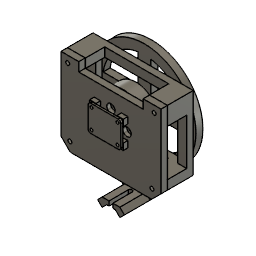
モータ取り付け台 (Autodesk Fusion 360 design; units mm, degrees)
Autodesk Fusion 360 part; units mm, degrees
sketch "スケッチ1" plane through (0, 0, 0) normal (0, 0, 1) x (1, 0, 0)
  line L0 (-38.8909, 38.8909) -> (0, 0)
  line L1 (0, 0) -> (38.8909, 38.8909)
  line L2 (38.8909, 38.8909) -> (-38.8909, 38.8909) construction
  line L3 (0, 38.8909) -> (0, 0) construction
  line L4 (-24.5921, 31.6632) -> (-3.3789, 10.45)
  line L5 (-3.3789, 10.45) -> (3.3789, 10.45)
  line L6 (3.3789, 10.45) -> (24.5921, 31.6632)
  line L7 (24.5921, 31.6632) -> (24.5921, 38.8909)
  line L8 (-24.5921, 38.8909) -> (-24.5921, 31.6632)
  line L9 (-24.5921, 38.8909) -> (24.5921, 38.8909)
  line L10 (-38.8909, 38.8909) -> (-38.8909, 45.9909)
  line L11 (-31.8909, 45.9909) -> (31.8909, 45.9909)
  line L12 (38.8909, 45.9909) -> (38.8909, 38.8909)
  line L13 (31.8909, 45.9909) -> (-31.8909, 45.9909)
  line L14 (-38.8909, 45.9909) -> (-38.8909, 95.9909)
  line L15 (-38.8909, 95.9909) -> (38.8909, 95.9909)
  line L16 (38.8909, 95.9909) -> (38.8909, 45.9909)
  line L17 (38.8909, 45.9909) -> (-38.8909, 95.9909) construction
  line L18 (-38.8909, 45.9909) -> (38.8909, 95.9909) construction
  line L19 (-31.8909, 45.9909) -> (-31.8909, 81.9198)
  line L20 (-24.8198, 88.9909) -> (24.8198, 88.9909)
  line L21 (31.8909, 81.9198) -> (31.8909, 45.9909)
  line L22 (-24.8198, 88.9909) -> (-31.8909, 81.9198)
  line L23 (24.8198, 88.9909) -> (31.8909, 81.9198)
  point P0 (0, 70.9909)
  point P1 (0, 70.9909)
  dimension "d1" = 55
  dimension "d3" = 55
  dimension "d4" = 5
  dimension "d5" = 5
  dimension "d6" = 30
  dimension "d7" = 30
  dimension "d8" = 10.45
  dimension "d9" = 7.1
  dimension "d10" = 50
  dimension "d11" = 7
  dimension "d13" = 45
  dimension "d14" = 45
  dimension "d15" = 10
  dimension "d16" = 10
  dimension "d17" = 7
  dimension "d18" = 7
  dimension "d19" = 57.1
  dimension "d20" = 7.1
  constraint coincident L0.end L1.start
  constraint horizontal L2
  constraint midpoint L2 L3.start
  constraint perpendicular L3 L5
  constraint parallel L0 L4
  constraint parallel L1 L6
  constraint perpendicular L0 L1
  constraint vertical L8
  constraint vertical L7
  constraint coincident L2 L8.start
  constraint coincident L2 L7.end
  constraint coincident L0.start L2.end
  constraint horizontal L11
  constraint vertical L10
  constraint vertical L12
  constraint horizontal L13
  constraint perpendicular L13 L14
  constraint parallel L13 L15
  constraint parallel L14 L16
  constraint coincident L17 P1
  constraint coincident L18 P1
  constraint coincident L10.end L14.start
  constraint coincident P1 P0
  measures "d1" distance of L0.end L1.end
  measures "d3" distance of L0.start L0.end
  measures "d4" distance of L1 L6
  measures "d5" distance of L0 L4
  measures "d6" distance of L5.end L6.end
  measures "d7" distance of L4.start L4.end
  measures "d8" distance of L0.end L5
  measures "d9" distance of L9 L11
  measures "d10" distance of L12.start L15.end
  measures "d11" distance of L16 L21
  measures "d13" angle of L20 L22
  measures "d14" angle of L20 L23
  measures "d15" distance of L20.start L19.end
  measures "d16" distance of L20.end L21.start
  measures "d17" distance of L15 L20
  measures "d18" distance of L14 L19
  measures "d19" distance of L9 L15
  measures "d20" distance of L0.start L10.end
extrude "押し出し1" add sketch "スケッチ1" along normal mid plane 5 makes body 1
sketch "スケッチ2" plane through (0, 0, 2.5) normal (0, 0, 1) x (1, 0, 0)
  line L0 (-31.8909, 81.9198) -> (-24.8198, 88.9909)
  line L1 (-24.8198, 88.9909) -> (24.8198, 88.9909)
  line L2 (24.8198, 88.9909) -> (31.8909, 81.9198)
  line L3 (31.8909, 81.9198) -> (31.8909, 45.9909)
  line L4 (31.8909, 45.9909) -> (-31.8909, 45.9909)
  line L5 (-31.8909, 45.9909) -> (-31.8909, 81.9198)
  line L6 (-3.3789, 10.45) -> (-24.5921, 31.6632)
  line L7 (-24.5921, 31.6632) -> (-24.5921, 38.8909)
  line L8 (-24.5921, 38.8909) -> (24.5921, 38.8909)
  line L9 (24.5921, 38.8909) -> (24.5921, 31.6632)
  line L10 (24.5921, 31.6632) -> (3.3789, 10.45)
  line L11 (3.3789, 10.45) -> (-3.3789, 10.45)
  line L12 (-38.8909, 38.8909) -> (0, 0)
  line L13 (0, 0) -> (38.8909, 38.8909)
  line L14 (38.8909, 38.8909) -> (38.8909, 95.9909)
  line L15 (38.8909, 95.9909) -> (-38.8909, 95.9909)
  line L16 (-38.8909, 95.9909) -> (-38.8909, 38.8909)
  line L17 (-24.8198, 95.9909) -> (-24.8198, 88.9909)
  line L18 (-24.8198, 88.9909) -> (-31.8909, 81.9198)
  line L19 (-31.8909, 81.9198) -> (-38.8909, 81.9198)
  line L20 (-38.8909, 81.9198) -> (-38.8909, 95.9909)
  line L21 (-38.8909, 95.9909) -> (-24.8198, 95.9909)
  line L22 (24.8198, 95.9909) -> (24.8198, 88.9909)
  line L23 (24.8198, 88.9909) -> (31.8909, 81.9198)
  line L24 (31.8909, 81.9198) -> (38.8909, 81.9198)
  line L25 (38.8909, 81.9198) -> (38.8909, 95.9909)
  line L26 (38.8909, 95.9909) -> (24.8198, 95.9909)
  line L27 (-24.5921, 45.9909) -> (-24.5921, 31.6632)
  line L28 (-24.5921, 31.6632) -> (-31.6632, 31.6632)
  line L29 (-31.6632, 31.6632) -> (-38.8909, 38.8909)
  line L30 (-38.8909, 38.8909) -> (-38.8909, 45.9909)
  line L31 (-38.8909, 45.9909) -> (-24.5921, 45.9909)
  line L32 (24.5921, 45.9909) -> (24.5921, 31.6632)
  line L33 (24.5921, 31.6632) -> (31.6632, 31.6632)
  line L34 (31.6632, 31.6632) -> (38.8909, 38.8909)
  line L35 (38.8909, 38.8909) -> (38.8909, 45.9909)
  line L36 (38.8909, 45.9909) -> (24.5921, 45.9909)
  line L37 (-3.3789, 10.45) -> (-6.9145, 6.9145)
  line L38 (-6.9145, 6.9145) -> (0, 0)
  line L39 (0, 0) -> (6.9145, 6.9145)
  line L40 (6.9145, 6.9145) -> (3.3789, 10.45)
  line L41 (3.3789, 10.45) -> (-3.3789, 10.45)
  constraint coincident L15 L17.start
  constraint coincident L0.end L1.start
  constraint perpendicular L1 L17
  constraint coincident L0.start L5.end
  constraint coincident L16 L19.end
  constraint perpendicular L16 L19
  constraint coincident L15.end L16.start
  constraint coincident L15 L22.start
  constraint coincident L1.end L2.start
  constraint coincident L2.end L3.start
  constraint coincident L14 L24.end
  constraint perpendicular L14 L24
  constraint coincident L14.end L15.start
  constraint vertical L22
  constraint coincident L4 L27.start
  constraint coincident L6.end L7.start
  constraint coincident L12 L28.end
  constraint perpendicular L27 L28
  constraint vertical L27
  constraint coincident L16 L30.end
  constraint coincident L12.start L16.end
  constraint horizontal L31
  constraint vertical L32
  constraint perpendicular L32 L33
  constraint perpendicular L33 L35
  constraint coincident L4 L32.start
  constraint coincident L9.end L10.start
  constraint coincident L13 L33.end
  constraint coincident L14 L35.end
  constraint coincident L13.end L14.start
  constraint horizontal L36
  constraint coincident L6.start L11.end
  constraint coincident L12 L37.end
  constraint perpendicular L12 L37
  constraint perpendicular L12 L39
  constraint coincident L10.end L11.start
  constraint coincident L13 L39.end
  constraint coincident L12.end L13.start
  constraint perpendicular L13 L40
extrude "押し出し2" add sketch "スケッチ2" along normal blind 15 contours L0 L15 L16 L17 L18 L19 L20 L21 | L4 L7 L12 L16 L27 L28 L29 L30 L31 | L2 L14 L15 L22 L23 L24 L25 L26 | L4 L9 L13 L14 L32 L33 L34 L35 L36 bodies 1
extrude "押し出し3" add sketch "スケッチ2" along normal blind 60 contours L11 L12 L13 L37 L38 L39 L40 L41 bodies 1
sketch "スケッチ3" plane through (0, 0, -2.5) normal (0, 0, -1) x (-1, 0, 0)
  line L0 (24.8198, 88.9909) -> (31.8909, 81.9198)
  line L1 (31.8909, 81.9198) -> (31.8909, 45.9909)
  line L2 (31.8909, 45.9909) -> (-31.8909, 45.9909)
  line L3 (-31.8909, 45.9909) -> (-31.8909, 81.9198)
  line L4 (-31.8909, 81.9198) -> (-24.8198, 88.9909)
  line L5 (-24.8198, 88.9909) -> (24.8198, 88.9909)
  line L6 (24.5921, 31.6632) -> (3.3789, 10.45)
  line L7 (3.3789, 10.45) -> (-3.3789, 10.45)
  line L8 (-3.3789, 10.45) -> (-24.5921, 31.6632)
  line L9 (-24.5921, 31.6632) -> (-24.5921, 38.8909)
  line L10 (-24.5921, 38.8909) -> (24.5921, 38.8909)
  line L11 (24.5921, 38.8909) -> (24.5921, 31.6632)
  line L12 (0, 0) -> (38.8909, 38.8909)
  line L13 (38.8909, 38.8909) -> (38.8909, 95.9909)
  line L14 (38.8909, 95.9909) -> (-38.8909, 95.9909)
  line L15 (-38.8909, 95.9909) -> (-38.8909, 38.8909)
  line L16 (-38.8909, 38.8909) -> (0, 0)
  line L17 (-38.8909, 95.9909) -> (-28.3553, 85.4553) construction
  line L18 (38.8909, 95.9909) -> (28.3553, 85.4553) construction
  circle A0 centre (-33.6231, 90.7231) radius 3.5
  circle A1 centre (33.6231, 90.7231) radius 3.5
  circle A2 centre (-31.8909, 38.8909) radius 3.5
  circle A3 centre (31.8909, 38.8909) radius 3.5
  line L19 (-24.5921, 38.8909) -> (-38.8909, 38.8909) construction
  line L20 (-31.8909, 45.9909) -> (-31.8909, 31.8909) construction
  line L21 (24.5921, 38.8909) -> (38.8909, 38.8909) construction
  line L22 (31.8909, 45.9909) -> (31.8909, 31.8909) construction
  circle A4 centre (-31.8909, 38.8909) radius 1.5
  circle A5 centre (31.8909, 38.8909) radius 1.5
  circle A6 centre (33.6231, 90.7231) radius 1.5
  circle A7 centre (-33.6231, 90.7231) radius 1.5
  dimension "d27" = 7
  dimension "d28" = 7
  dimension "d29" = 7
  dimension "d30" = 7
  dimension "d31" = 3
  dimension "d32" = 3
  dimension "d33" = 3
  dimension "d34" = 3
  constraint coincident L14.end L15.start
  constraint midpoint L4 L17.end
  constraint coincident L13.end L14.start
  constraint midpoint L0 L18.end
  constraint midpoint L17 A0.centre
  constraint midpoint L18 A1.centre
  constraint coincident L9.end L10.start
  constraint coincident L15.end L16.start
  constraint coincident L2.end L3.start
  constraint coincident L16 L20.end
  constraint perpendicular L19 L20
  constraint coincident A2.centre L19
  constraint coincident A2.centre L20
  constraint coincident L10.end L11.start
  constraint coincident L12.end L13.start
  constraint coincident L1.end L2.start
  constraint coincident L12 L22.end
  constraint perpendicular L21 L22
  constraint coincident A3.centre L22
  constraint coincident A3.centre L21
  constraint concentric A2 A4
  constraint concentric A3 A5
  constraint concentric A1 A6
  constraint concentric A0 A7
  measures "d27" diameter of A0
  measures "d28" diameter of A1
  measures "d29" diameter of A2
  measures "d30" diameter of A3
  measures "d31" diameter of A4
  measures "d32" diameter of A5
  measures "d33" diameter of A6
  measures "d34" diameter of A7
extrude "押し出し4" cut sketch "スケッチ3" against normal blind 25 contours A4 | A5 | A6 | A7 bodies 1
extrude "押し出し7" cut 1 faces at (0, 6.9667, 62.5) along direction (0, 0, -1) blind 65 on bodies 1 bodies 1
sketch "スケッチ8" plane through (0, 0, 2.5) normal (0, 0, 1) x (1, 0, 0)
  line L0 (-6.9145, 6.9145) -> (-3.3789, 10.45)
  line L1 (-3.3789, 10.45) -> (-24.5921, 31.6632)
  line L2 (-24.5921, 31.6632) -> (-31.6632, 31.6632)
  line L3 (-31.6632, 31.6632) -> (-6.9145, 6.9145)
  line L4 (3.3789, 10.45) -> (6.9145, 6.9145)
  line L5 (24.5921, 31.6632) -> (3.3789, 10.45)
  line L6 (6.9145, 6.9145) -> (31.6632, 31.6632)
  line L7 (-3.3789, 10.45) -> (3.3789, 10.45)
  line L8 (-6.9145, 13.9855) -> (6.9145, 13.9855)
  line L9 (6.9145, 13.9855) -> (10.45, 10.45)
  line L10 (-6.9145, 13.9855) -> (-10.45, 10.45)
  dimension "d52" = 5
  dimension "d53" = 5
  constraint coincident L0.end L1.start
  constraint coincident L4.start L5.end
  constraint coincident L1 L8.start
  constraint coincident L5 L8.end
  constraint coincident L6 L9.end
  constraint coincident L3 L10.end
  constraint perpendicular L1 L10
  constraint perpendicular L6 L9
  measures "d52" distance of L0 L10
  measures "d53" distance of L4 L9
extrude "押し出し9" add sketch "スケッチ8" against normal blind 5 contours L1 L5 L7 L8 bodies 1
extrude "押し出し10" add sketch "スケッチ8" along normal blind 20 contours L0 L1 L3 L10 | L1 L5 L7 L8 | L4 L5 L6 L9 bodies 1
sketch "スケッチ9" plane through (0, 10.45, 0) normal (0, -1, 0) x (1, 0, 0)
  line L0 (-3.3789, 22.5) -> (-3.3789, -2.5)
  line L1 (-3.3789, -2.5) -> (3.3789, -2.5)
  line L2 (3.3789, -2.5) -> (3.3789, 22.5)
  line L3 (3.3789, 22.5) -> (-3.3789, 22.5)
  arc A0 (-1.5, 7.5) -> (1.5, 7.5) centre (0, 7.5) ccw
  line L4 (0, 7.5) -> (0, -2.5) construction
  line L5 (-1.5, 7.5) -> (-1.5, 22.5)
  line L6 (1.5, 22.5) -> (1.5, 7.5)
  dimension "d58" = 10
  dimension "d59" = 1.5
  constraint coincident A0.centre L4.start
  constraint midpoint L1 L4.end
  constraint vertical L4
  constraint coincident L3 L5.end
  constraint tangent A0 L5
  constraint coincident L3 L6.start
  constraint tangent A0 L6
  constraint vertical L6
  constraint vertical L5
  measures "d58" distance of A0.centre L4.end
  measures "d59" radius of A0
extrude "押し出し11" cut sketch "スケッチ9" against normal blind 4 contours L3 A0 L5 L6 bodies 1
extrude "押し出し12" add sketch "スケッチ3" against normal blind 4 contours A4 | A5 | A6 | A7 bodies 1
sketch "スケッチ10" plane through (0, 0, 17.5) normal (0, 0, 1) x (1, 0, 0)
  circle A0 centre (-31.8909, 38.8909) radius 1.5
  line L0 (-38.8909, 45.9909) -> (-38.8909, 38.8909)
  line L1 (-38.8909, 38.8909) -> (-31.6632, 31.6632)
  line L2 (-31.6632, 31.6632) -> (-24.5921, 31.6632)
  line L3 (-24.5921, 31.6632) -> (-24.5921, 45.9909)
  line L4 (-24.5921, 45.9909) -> (-38.8909, 45.9909)
  line L5 (-38.8909, 95.9909) -> (-38.8909, 81.9198)
  line L6 (31.6632, 31.6632) -> (38.8909, 38.8909)
  line L7 (38.8909, 81.9198) -> (38.8909, 95.9909)
  line L8 (-38.8909, 95.9909) -> (-38.8909, 38.8909)
  line L9 (-38.8909, 38.8909) -> (-31.6632, 31.6632)
  line L10 (-31.6632, 31.6632) -> (31.6632, 31.6632)
  line L11 (31.6632, 31.6632) -> (38.8909, 38.8909)
  line L12 (38.8909, 38.8909) -> (38.8909, 95.9909)
  line L13 (38.8909, 95.9909) -> (-38.8909, 95.9909)
  line L14 (31.8909, 45.9909) -> (31.8909, 81.9198)
  line L15 (31.8909, 81.9198) -> (24.8198, 88.9909)
  line L16 (6.9145, 13.9855) -> (24.5921, 31.6632)
  line L17 (24.5921, 31.6632) -> (24.5921, 38.8909)
  line L18 (24.5921, 38.8909) -> (-24.5921, 38.8909)
  line L19 (-24.5921, 38.8909) -> (-24.5921, 31.6632)
  line L20 (-24.5921, 31.6632) -> (-6.9145, 13.9855)
  line L21 (-6.9145, 13.9855) -> (6.9145, 13.9855)
  line L22 (3.3789, 10.45) -> (-3.3789, 10.45)
  line L23 (-3.3789, 10.45) -> (-6.9145, 6.9145)
  line L24 (-6.9145, 6.9145) -> (-38.8909, 38.8909)
  line L25 (-38.8909, 38.8909) -> (-38.8909, 95.9909)
  line L26 (-38.8909, 95.9909) -> (38.8909, 95.9909)
  line L27 (38.8909, 95.9909) -> (38.8909, 38.8909)
  line L28 (38.8909, 38.8909) -> (6.9145, 6.9145)
  line L29 (6.9145, 6.9145) -> (3.3789, 10.45)
  line L30 (-24.8198, 88.9909) -> (-31.8909, 81.9198)
  line L31 (-31.8909, 81.9198) -> (-31.8909, 45.9909)
  line L32 (-31.8909, 45.9909) -> (31.8909, 45.9909)
  line L33 (31.8909, 45.9909) -> (31.8909, 81.9198)
  line L34 (31.8909, 81.9198) -> (24.8198, 88.9909)
  line L35 (24.8198, 88.9909) -> (-24.8198, 88.9909)
  line L36 (0, 88.9909) -> (0, 45.9909) construction
  circle A1 centre (0, 76.9909) radius 1.5
  circle A2 centre (12.5, 67.4909) radius 1.5
  circle A3 centre (0, 57.9909) radius 1.5
  circle A4 centre (-12.5, 67.4909) radius 1.5
  line L37 (-12.5, 67.4909) -> (12.5, 67.4909) construction
  line L38 (0, 76.9909) -> (0, 57.9909) construction
  circle A5 centre (31.8909, 38.8909) radius 1.5
  circle A6 centre (33.6231, 90.7231) radius 1.5
  circle A7 centre (-33.6231, 90.7231) radius 1.5
  circle A8 centre (-33.6231, 90.7231) radius 1.5
  circle A9 centre (33.6231, 90.7231) radius 1.5
  circle A10 centre (31.8909, 38.8909) radius 1.5
  circle A11 centre (0, 67.4909) radius 4
  point P0 (0, 67.4909)
  dimension "d64" = 3
  dimension "d65" = 3
  dimension "d66" = 3
  dimension "d67" = 3
  dimension "d68" = 19
  dimension "d69" = 25
  dimension "d70" = 12.5
  dimension "d71" = 9.5
  dimension "d78" = 3
  dimension "d79" = 3
  dimension "d80" = 3
  dimension "d81" = 8
  constraint coincident L5.start L8.start
  constraint coincident L0.end L1.start
  constraint coincident L1.end L2.start
  constraint coincident L6.start L10.end
  constraint coincident L6.end L11.end
  constraint coincident L7.end L12.end
  constraint midpoint L35 L36.start
  constraint midpoint L32 L36.end
  constraint midpoint L36 P0
  constraint coincident A4.centre L37.start
  constraint coincident A2.centre L37.end
  constraint coincident A1.centre L38.start
  constraint coincident A3.centre L38.end
  constraint coincident P0 L37
  constraint coincident P0 L38
  constraint vertical L38
  constraint horizontal L37
  constraint concentric A7 A8
  constraint concentric A6 A9
  constraint concentric A5 A10
  constraint coincident P0 A11.centre
  measures "d64" diameter of A1
  measures "d65" diameter of A3
  measures "d66" diameter of A4
  measures "d67" diameter of A2
  measures "d68" distance of A1.centre A3.centre
  measures "d69" distance of A2.centre A4.centre
  measures "d70" distance of P0 A2.centre
  measures "d71" distance of P0 A1.centre
  measures "d78" diameter of A10
  measures "d79" diameter of A9
  measures "d80" diameter of A8
  measures "d81" diameter of A11
extrude "押し出し13" add sketch "スケッチ10" along normal blind 5 separate body contours L0 L1 L2 L3 L4 L8 L9 L10 L19 L24 L25 L32 | L3 L4 L5 L6 L7 L8 L10 L11 L12 L13 L14 L15 L17 L18 L25 L26 L27 L28 L30 L31 L32 L33 L34 L35 | L4 L14 L15 L30 L31 L32 L33 L34 L35 | L3 L10 L17 L18 L19 makes body 2
sketch "スケッチ11" plane through (0, 0, 22.5) normal (0, 0, 1) x (1, 0, 0)
  circle A0 centre (-12.5, 67.4909) radius 1.5
  circle A1 centre (0, 76.9909) radius 1.5
  circle A2 centre (0, 57.9909) radius 1.5
  circle A3 centre (12.5, 67.4909) radius 1.5
  line L0 (-31.6632, 31.6632) -> (31.6632, 31.6632)
  line L1 (31.6632, 31.6632) -> (38.8909, 38.8909)
  line L2 (38.8909, 38.8909) -> (38.8909, 95.9909)
  line L3 (38.8909, 95.9909) -> (-38.8909, 95.9909)
  line L4 (-38.8909, 95.9909) -> (-38.8909, 38.8909)
  line L5 (-38.8909, 38.8909) -> (-31.6632, 31.6632)
  line L6 (25, 95.9909) -> (-25, 95.9909)
  line L7 (-25, 95.9909) -> (-25, 88.9909)
  line L8 (-25, 88.9909) -> (25, 88.9909)
  line L9 (25, 88.9909) -> (25, 95.9909)
  line L10 (25, 95.9909) -> (-25, 88.9909) construction
  line L11 (-25, 95.9909) -> (25, 88.9909) construction
  line L12 (0, 76.9909) -> (0, 92.4909) construction
  circle A4 centre (-31.8909, 38.8909) radius 1.5
  circle A5 centre (31.8909, 38.8909) radius 1.5
  circle A6 centre (33.6231, 90.7231) radius 1.5
  circle A7 centre (-33.6231, 90.7231) radius 1.5
  circle A8 centre (0, 67.4909) radius 4
  point P0 (0, 92.4909)
  dimension "d74" = 50
  dimension "d75" = 7
  constraint horizontal L6
  constraint perpendicular L6 L7
  constraint parallel L6 L8
  constraint parallel L7 L9
  constraint coincident L10 P0
  constraint coincident L11 P0
  constraint coincident L3 L6.start
  constraint coincident A1.centre L12.start
  constraint coincident P0 L12.end
  constraint vertical L12
  measures "d74" distance of L7.end L8.end
  measures "d75" distance of L6.start L8.end
extrude "押し出し14" cut sketch "スケッチ11" against normal blind 5 contours L3 L6 L7 L8 L9 bodies 2
sketch "スケッチ12" plane through (0, 0, 17.5) normal (0, 0, -1) x (-1, 0, 0)
  line L0 (25, 95.9909) -> (25, 88.9909)
  line L1 (25, 88.9909) -> (-25, 88.9909)
  line L2 (-25, 88.9909) -> (-25, 95.9909)
  line L3 (-25, 95.9909) -> (-38.8909, 95.9909)
  line L4 (-38.8909, 95.9909) -> (-38.8909, 38.8909)
  line L5 (-38.8909, 38.8909) -> (-31.6632, 31.6632)
  line L6 (-31.6632, 31.6632) -> (31.6632, 31.6632)
  line L7 (31.6632, 31.6632) -> (38.8909, 38.8909)
  line L8 (38.8909, 38.8909) -> (38.8909, 95.9909)
  line L9 (38.8909, 95.9909) -> (25, 95.9909)
  circle A0 centre (-12.5, 67.4909) radius 1.5
  circle A1 centre (0, 57.9909) radius 1.5
  circle A2 centre (33.6231, 90.7231) radius 1.5
  circle A3 centre (0, 67.4909) radius 4
  circle A4 centre (-31.8909, 38.8909) radius 1.5
  circle A5 centre (31.8909, 38.8909) radius 1.5
  circle A6 centre (12.5, 67.4909) radius 1.5
  circle A7 centre (-33.6231, 90.7231) radius 1.5
  circle A8 centre (0, 76.9909) radius 1.5
  circle A9 centre (0, 67.4909) radius 16.25
  dimension "d82" = 32.5
  constraint concentric A3 A9
  measures "d82" diameter of A9
extrude "押し出し15" add sketch "スケッチ12" along normal blind 1.5 separate body contours A9 makes body 3
sketch "スケッチ13" plane through (0, 0, 16) normal (0, 0, -1) x (-1, 0, 0)
  circle A0 centre (0, 76.9909) radius 1.5
  circle A1 centre (0, 67.4909) radius 4
  circle A2 centre (0, 57.9909) radius 1.5
  circle A3 centre (12.5, 67.4909) radius 1.5
  circle A4 centre (-12.5, 67.4909) radius 1.5
  circle A5 centre (0, 67.4909) radius 16.25
  circle A6 centre (0, 67.4909) radius 7.5
  dimension "d85" = 15
  constraint concentric A1 A6
  measures "d85" diameter of A6
extrude "押し出し16" add sketch "スケッチ13" along normal blind 3 contours A6 bodies 3
sketch "スケッチ15" plane through (0, 0, 13) normal (0, 0, -1) x (-1, 0, 0)
  circle A0 centre (0, 67.4909) radius 4
  circle A1 centre (0, 67.4909) radius 7.5
  circle A2 centre (0, 67.4909) radius 17.5
  dimension "d88" = 35
  constraint concentric A0 A2
  measures "d88" diameter of A2
extrude "押し出し17" add sketch "スケッチ15" along normal blind 9 contours A0 | A1 | A2 bodies 3
sketch "スケッチ16" plane through (0, 0, 13) normal (0, 0, 1) x (1, 0, 0)
  circle A0 centre (0, 67.4909) radius 4
  circle A1 centre (0, 67.4909) radius 3.25
  dimension "d91" = 6.5
  constraint concentric A0 A1
  measures "d91" diameter of A1
extrude "押し出し18" add sketch "スケッチ16" along normal blind 7 contours A1 bodies 3
sketch "スケッチ17" plane through (0, 0, 0) normal (1, 0, 0) x (0, 0, -1)
  line L0 (-4, 49.9909) -> (-4, 84.9909)
  line L1 (-4, 84.9909) -> (-3, 84.9909)
  line L2 (-18, 67.4909) -> (2, 67.4909)
  line L3 (-1, 67.4909) -> (-4, 67.4909)
  line L4 (-4, 84.9909) -> (-4, 67.4909)
  line L5 (-20, 70.7409) -> (-20, 64.2409)
  line L6 (-3, 84.9909) -> (-1, 74.4909)
  line L7 (-1, 74.4909) -> (-1, 67.4909)
  dimension "d94" = 19
  dimension "d95" = 1
  dimension "d96" = 7
  constraint coincident L0.end L1.start
  constraint perpendicular L0 L1
  constraint coincident L3.start L2
  constraint midpoint L0 L3.end
  constraint vertical L7
  measures "d94" distance of L3.start L5
  measures "d95" distance of L0.end L1.end
  measures "d96" distance of L3.start L6.end
revolve "回転1" add sketch "スケッチ17" angle 360 about axis through (0, 67.4909, 18) along (0, 0, -1) bodies 3
sketch "スケッチ18" plane through (0, 0, 1) normal (0, 0, -1) x (-1, 0, 0)
  circle A0 centre (0, 67.4909) radius 7
  circle A1 centre (0, 67.4909) radius 2
  dimension "d98" = 4
  constraint concentric A0 A1
  measures "d98" diameter of A1
extrude "押し出し19" add sketch "スケッチ18" along normal blind 9.1 contours A1 bodies 3
sketch "スケッチ19" plane through (0, 0, -2.5) normal (0, 0, -1) x (-1, 0, 0)
  line L0 (-6.9145, 13.9855) -> (-24.5921, 31.6632)
  line L1 (-24.5921, 31.6632) -> (-24.5921, 38.8909)
  line L2 (-24.5921, 38.8909) -> (24.5921, 38.8909)
  line L3 (24.5921, 38.8909) -> (24.5921, 31.6632)
  line L4 (24.5921, 31.6632) -> (6.9145, 13.9855)
  line L5 (6.9145, 13.9855) -> (-6.9145, 13.9855)
  line L6 (-3.3789, 10.45) -> (3.3789, 10.45)
  line L7 (3.3789, 10.45) -> (6.9145, 6.9145)
  line L8 (6.9145, 6.9145) -> (38.8909, 38.8909)
  line L9 (38.8909, 38.8909) -> (38.8909, 95.9909)
  line L10 (38.8909, 95.9909) -> (-38.8909, 95.9909)
  line L11 (-38.8909, 95.9909) -> (-38.8909, 38.8909)
  line L12 (-38.8909, 38.8909) -> (-6.9145, 6.9145)
  line L13 (-6.9145, 6.9145) -> (-3.3789, 10.45)
  line L14 (24.8198, 88.9909) -> (31.8909, 81.9198)
  line L15 (31.8909, 81.9198) -> (31.8909, 45.9909)
  line L16 (31.8909, 45.9909) -> (-31.8909, 45.9909)
  line L17 (-31.8909, 45.9909) -> (-31.8909, 81.9198)
  line L18 (-31.8909, 81.9198) -> (-24.8198, 88.9909)
  line L19 (-24.8198, 88.9909) -> (24.8198, 88.9909)
  circle A0 centre (0, 67.4909) radius 2
  circle A1 centre (0, 67.4909) radius 2
  circle A2 centre (0, 67.4909) radius 40
  circle A3 centre (0, 67.4909) radius 10
  circle A4 centre (0, 67.4909) radius 3.75
  circle A5 centre (0, 67.4909) radius 32.5
  line L20 (-5, 99.604) -> (-5, 76.1511)
  line L21 (5, 99.604) -> (5, 76.1511)
  line L22 (8.6603, 72.4909) -> (32.1131, 72.4909)
  line L23 (8.6603, 62.4909) -> (32.1131, 62.4909)
  line L24 (5, 58.8306) -> (5, 35.3778)
  line L25 (-5, 58.8306) -> (-5, 35.3778)
  line L26 (-8.6603, 62.4909) -> (-32.1131, 62.4909)
  line L27 (-8.6603, 72.4909) -> (-32.1131, 72.4909)
  dimension "d101" = 4
  dimension "d102" = 80
  dimension "d103" = 20
  dimension "d104" = 7.5
  dimension "d107" = 65
  dimension "d108" = 10
  dimension "d109" = 10
  dimension "d110" = 10
  dimension "d111" = 10
  dimension "d112" = 5
  dimension "d113" = 5
  dimension "d114" = 5
  dimension "d115" = 5
  constraint concentric A0 A1
  constraint concentric A0 A2
  constraint concentric A1 A3
  constraint concentric A3 A4
  constraint concentric A1 A5
  constraint coincident A5 L20.start
  constraint coincident A3 L20.end
  constraint perpendicular L19 L20
  constraint coincident A5 L21.start
  constraint coincident A3 L21.end
  constraint perpendicular L19 L21
  constraint coincident A3 L22.start
  constraint coincident A5 L22.end
  constraint perpendicular L15 L22
  constraint coincident A3 L23.start
  constraint coincident A3 L24.start
  constraint coincident A5 L24.end
  constraint perpendicular L2 L24
  constraint coincident A3 L25.start
  constraint coincident A5 L25.end
  constraint coincident A3 L26.start
  constraint coincident A5 L26.end
  constraint coincident A3 L27.start
  constraint coincident A5 L27.end
  constraint coincident A5 L23.end
  constraint horizontal L27
  constraint horizontal L26
  constraint horizontal L23
  constraint vertical L25
  measures "d101" diameter of A1
  measures "d102" diameter of A2
  measures "d103" diameter of A3
  measures "d104" diameter of A4
  measures "d107" diameter of A5
  measures "d108" distance of L22 L23
  measures "d109" distance of L20 L21
  measures "d110" distance of L26 L27
  measures "d111" distance of L24 L25
  measures "d112" distance of A0.centre L27
  measures "d113" distance of A0.centre L21
  measures "d114" distance of A0.centre L22
  measures "d115" distance of A0.centre L24
extrude "押し出し20" add sketch "スケッチ19" against normal blind 3.5 separate body contours A4 makes body 4
extrude "押し出し21" add sketch "スケッチ19" along normal blind 6.5 contours L1 L2 L10 L11 L16 L17 L18 L19 A2 A5 | L1 L2 L3 A2 A5 | L11 A2 | L2 L3 L9 L10 L14 L15 L16 L19 A2 A5 | L9 A2 | L2 L16 L24 L25 | L2 A5 L24 L25 | L16 L17 A5 | L10 A2 A5 | L16 A3 L24 L25 | L15 L16 A5 | A3 | L17 A5 L26 L27 | L17 A3 L26 L27 | L10 A5 L20 L21 | L10 L19 L20 L21 | L17 L18 L19 A5 | L19 A3 L20 L21 | L14 L15 L19 A5 | L15 A3 L22 L23 | L15 A5 L22 L23 | A4 bodies 4
extrude "押し出し22" cut 1 faces at (24.2955, 69.1575, -2.5) along direction (0, 0, -1) blind 1 on bodies 4 bodies 4
sketch "スケッチ20" plane through (0, 0, -9) normal (0, 0, -1) x (-1, 0, 0)
  circle A0 centre (0, 67.4909) radius 2
  line L0 (32.1131, 72.4909) -> (8.6603, 72.4909)
  arc A1 (8.6603, 72.4909) -> (5, 76.1511) centre (0, 67.4909) ccw
  line L1 (5, 76.1511) -> (5, 99.604)
  arc A2 (32.1131, 72.4909) -> (5, 99.604) centre (0, 67.4909) ccw
  arc A3 (-5, 99.604) -> (-32.1131, 72.4909) centre (0, 67.4909) ccw
  line L2 (-5, 99.604) -> (-5, 76.1511)
  arc A4 (-5, 76.1511) -> (-8.6603, 72.4909) centre (0, 67.4909) ccw
  line L3 (-8.6603, 72.4909) -> (-32.1131, 72.4909)
  arc A5 (5, 58.8306) -> (8.6603, 62.4909) centre (0, 67.4909) ccw
  line L4 (8.6603, 62.4909) -> (32.1131, 62.4909)
  arc A6 (5, 35.3778) -> (32.1131, 62.4909) centre (0, 67.4909) ccw
  line L5 (5, 35.3778) -> (5, 58.8306)
  arc A7 (-8.6603, 62.4909) -> (-5, 58.8306) centre (0, 67.4909) ccw
  line L6 (-5, 58.8306) -> (-5, 35.3778)
  arc A8 (-32.1131, 62.4909) -> (-5, 35.3778) centre (0, 67.4909) ccw
  line L7 (-32.1131, 62.4909) -> (-8.6603, 62.4909)
  circle A9 centre (0, 67.4909) radius 40
  circle A10 centre (0, 67.4909) radius 2
  dimension "d120" = 4
  constraint concentric A0 A10
  measures "d120" diameter of A10
extrude "押し出し23" add sketch "スケッチ20" against normal blind 0.9 contours A0 A10 bodies 4
sketch "スケッチ21" plane through (0, 0, 22.5) normal (0, 0, 1) x (1, 0, 0)
  circle A0 centre (12.5, 67.4909) radius 1.5
  circle A1 centre (0, 57.9909) radius 1.5
  circle A2 centre (-33.6231, 90.7231) radius 1.5
  circle A3 centre (0, 67.4909) radius 4
  circle A4 centre (31.8909, 38.8909) radius 1.5
  circle A5 centre (-31.8909, 38.8909) radius 1.5
  circle A6 centre (-12.5, 67.4909) radius 1.5
  circle A7 centre (33.6231, 90.7231) radius 1.5
  circle A8 centre (0, 76.9909) radius 1.5
  line L0 (-25, 88.9909) -> (-25, 95.9909)
  line L1 (-25, 95.9909) -> (-38.8909, 95.9909)
  line L2 (-38.8909, 95.9909) -> (-38.8909, 38.8909)
  line L3 (-38.8909, 38.8909) -> (-31.6632, 31.6632)
  line L4 (-31.6632, 31.6632) -> (31.6632, 31.6632)
  line L5 (31.6632, 31.6632) -> (38.8909, 38.8909)
  line L6 (38.8909, 38.8909) -> (38.8909, 95.9909)
  line L7 (38.8909, 95.9909) -> (25, 95.9909)
  line L8 (25, 95.9909) -> (25, 88.9909)
  line L9 (25, 88.9909) -> (-25, 88.9909)
  circle A9 centre (0, 76.9909) radius 3.25
  circle A10 centre (12.5, 67.4909) radius 3.25
  circle A11 centre (-12.5, 67.4909) radius 3.25
  circle A12 centre (0, 57.9909) radius 3.25
  dimension "d123" = 6.5
  dimension "d124" = 6.5
  dimension "d125" = 6.5
  dimension "d126" = 6.5
  constraint concentric A8 A9
  constraint concentric A0 A10
  constraint concentric A6 A11
  constraint concentric A1 A12
  measures "d123" diameter of A9
  measures "d124" diameter of A10
  measures "d125" diameter of A11
  measures "d126" diameter of A12
extrude "押し出し24" cut sketch "スケッチ21" against normal blind 3 contours A9 | A10 | A11 | A12 bodies 2
ref_plane "作業平面1" through (0, 63.827, 26) normal (0, 0, 1) x (1, 0, 0)
sketch "スケッチ22" plane through (0, 0, 26) normal (0, 0, 1) x (1, 0, 0)
  circle A0 centre (0, 67.4909) radius 3.25
  line L0 (10.7, 57.3309) -> (-10.7, 57.3309)
  line L1 (-12.7, 59.3309) -> (-12.7, 75.6509)
  line L2 (-10.7, 77.6509) -> (10.7, 77.6509)
  line L3 (12.7, 75.6509) -> (12.7, 59.3309)
  line L4 (12.7, 57.3309) -> (-12.7, 77.6509) construction
  line L5 (-12.7, 57.3309) -> (12.7, 77.6509) construction
  circle A1 centre (-10.1, 75.0509) radius 1.1
  circle A2 centre (10.1, 75.0509) radius 1.1
  circle A3 centre (-10.1, 59.9309) radius 1.1
  circle A4 centre (10.1, 59.9309) radius 1.1
  arc A5 (-10.7, 77.6509) -> (-12.7, 75.6509) centre (-10.7, 75.6509) ccw
  arc A6 (12.7, 75.6509) -> (10.7, 77.6509) centre (10.7, 75.6509) ccw
  arc A7 (10.7, 57.3309) -> (12.7, 59.3309) centre (10.7, 59.3309) ccw
  arc A8 (-12.7, 59.3309) -> (-10.7, 57.3309) centre (-10.7, 59.3309) ccw
  point P0 (0, 67.4909)
  dimension "d130" = 20.32
  dimension "d131" = 25.4
  dimension "d132" = 2.2
  dimension "d133" = 2.2
  dimension "d134" = 2.2
  dimension "d135" = 2.2
  dimension "d136" = 2.6
  dimension "d137" = 2.6
  dimension "d138" = 2.6
  dimension "d139" = 2.6
  dimension "d140" = 2.6
  dimension "d141" = 2.6
  dimension "d142" = 2.6
  dimension "d143" = 2.6
  dimension "d144" = 2
  constraint horizontal L0
  constraint perpendicular L0 L1
  constraint parallel L0 L2
  constraint parallel L1 L3
  constraint coincident L4 P0
  constraint coincident L5 P0
  constraint coincident P0 A0.centre
  constraint coincident L4.end L2
  constraint coincident L4.end L1
  constraint tangent L2 A5
  constraint tangent L1 A5
  constraint coincident L5.end L2
  constraint coincident L5.end L3
  constraint tangent L2 A6
  constraint tangent L3 A6
  constraint equal A5 A6
  constraint coincident L4.start L0
  constraint coincident L4.start L3
  constraint tangent L0 A7
  constraint tangent L3 A7
  constraint equal A5 A7
  constraint coincident L5.start L1
  constraint coincident L5.start L0
  constraint tangent L1 A8
  constraint tangent L0 A8
  constraint equal A5 A8
  measures "d130" distance of L5.start L4.end
  measures "d131" distance of L4.end L5.end
  measures "d132" diameter of A1
  measures "d133" diameter of A2
  measures "d134" diameter of A3
  measures "d135" diameter of A4
  measures "d136" distance of L3 A4.centre
  measures "d137" distance of L1 A3.centre
  measures "d138" distance of L3 A2.centre
  measures "d139" distance of L1 A1.centre
  measures "d140" distance of L2 A1.centre
  measures "d141" distance of L2 A2.centre
  measures "d142" distance of L0 A4.centre
  measures "d143" distance of L0 A3.centre
  measures "d144" radius of A5
extrude "押し出し25" add sketch "スケッチ22" along normal blind 1.5 separate body contours A0 | L0 L1 L2 L3 A5 A6 A7 A8 makes body 5
sketch "スケッチ23" plane through (0, 0, 26) normal (0, 0, -1) x (-1, 0, 0)
  circle A0 centre (10.1, 59.9309) radius 1.1
  circle A1 centre (-10.1, 75.0509) radius 1.1
  circle A2 centre (-10.1, 59.9309) radius 1.1
  circle A3 centre (10.1, 75.0509) radius 1.1
  arc A4 (12.7, 75.6509) -> (10.7, 77.6509) centre (10.7, 75.6509) ccw
  line L0 (10.7, 77.6509) -> (-10.7, 77.6509)
  arc A5 (-10.7, 77.6509) -> (-12.7, 75.6509) centre (-10.7, 75.6509) ccw
  line L1 (-12.7, 75.6509) -> (-12.7, 59.3309)
  arc A6 (-12.7, 59.3309) -> (-10.7, 57.3309) centre (-10.7, 59.3309) ccw
  line L2 (-10.7, 57.3309) -> (10.7, 57.3309)
  arc A7 (10.7, 57.3309) -> (12.7, 59.3309) centre (10.7, 59.3309) ccw
  line L3 (12.7, 59.3309) -> (12.7, 75.6509)
  line L4 (-8.1, 75.0509) -> (-8.1, 78.0509)
  line L5 (-8.1, 78.0509) -> (-13.1, 78.0509)
  line L6 (-13.1, 78.0509) -> (-13.1, 73.0509)
  line L7 (-13.1, 73.0509) -> (-10.1, 73.0509)
  arc A8 (-10.1, 73.0509) -> (-8.1, 75.0509) centre (-10.1, 75.0509) ccw
  line L8 (-10.1, 61.9309) -> (-13.1, 61.9309)
  line L9 (-13.1, 61.9309) -> (-13.1, 56.9309)
  line L10 (-13.1, 56.9309) -> (-8.1, 56.9309)
  line L11 (-8.1, 56.9309) -> (-8.1, 59.9309)
  line L12 (8.1, 75.0509) -> (8.1, 78.0509)
  line L13 (8.1, 78.0509) -> (13.1, 78.0509)
  line L14 (13.1, 78.0509) -> (13.1, 73.0509)
  line L15 (13.1, 73.0509) -> (10.1, 73.0509)
  line L16 (10.1, 61.9309) -> (13.1, 61.9309)
  line L17 (13.1, 61.9309) -> (13.1, 56.9309)
  line L18 (13.1, 56.9309) -> (8.1, 56.9309)
  line L19 (8.1, 56.9309) -> (8.1, 59.9309)
  arc A9 (8.1, 75.0509) -> (10.1, 73.0509) centre (10.1, 75.0509) ccw
  arc A10 (10.1, 61.9309) -> (8.1, 59.9309) centre (10.1, 59.9309) ccw
  arc A11 (-8.1, 59.9309) -> (-10.1, 61.9309) centre (-10.1, 59.9309) ccw
  circle A12 centre (-10.1, 75.0509) radius 1.05
  circle A13 centre (10.1, 75.0509) radius 1.05
  circle A14 centre (10.1, 59.9309) radius 1.05
  circle A15 centre (-10.1, 59.9309) radius 1.05
  dimension "d147" = 4
  dimension "d149" = 4
  dimension "d150" = 4
  dimension "d151" = 4
  dimension "d152" = 3
  dimension "d153" = 3
  dimension "d154" = 3
  dimension "d155" = 3
  dimension "d156" = 3
  dimension "d157" = 3
  dimension "d159" = 3
  dimension "d160" = 3
  dimension "d161" = 2.1
  dimension "d162" = 2.1
  dimension "d163" = 2.1
  dimension "d164" = 2.1
  constraint concentric A3 A9
  constraint concentric A0 A10
  constraint concentric A1 A8
  constraint concentric A2 A11
  constraint tangent L7 A8
  constraint tangent L4 A8
  constraint vertical L6
  constraint horizontal L7
  constraint vertical L4
  constraint horizontal L5
  constraint tangent L11 A11
  constraint tangent L8 A11
  constraint horizontal L8
  constraint vertical L11
  constraint horizontal L10
  constraint vertical L9
  constraint tangent L15 A9
  constraint tangent L16 A10
  constraint tangent L19 A10
  constraint tangent L12 A9
  constraint horizontal L15
  constraint vertical L12
  constraint horizontal L13
  constraint vertical L14
  constraint horizontal L16
  constraint vertical L19
  constraint horizontal L18
  constraint vertical L17
  constraint concentric A8 A12
  constraint concentric A9 A13
  constraint concentric A10 A14
  constraint concentric A11 A15
  measures "d147" diameter of A9
  measures "d149" diameter of A10
  measures "d150" diameter of A8
  measures "d151" diameter of A11
  measures "d152" distance of L4.start L4.end
  measures "d153" distance of L6.end L7.end
  measures "d154" horizontal distance of L8.start L8.end
  measures "d155" distance of L10.end L11.end
  measures "d156" distance of L16.start L16.end
  measures "d157" distance of L18.end L19.end
  measures "d159" distance of L14.end L15.end
  measures "d160" distance of L12.start L12.end
  measures "d161" diameter of A12
  measures "d162" diameter of A13
  measures "d163" diameter of A14
  measures "d164" diameter of A15
extrude "押し出し26" add sketch "スケッチ23" along normal blind 3.5 contours A4 L0 L3 L12 L15 A9 | A4 L0 L3 L12 L13 L14 L15 | L2 A7 L3 L16 L17 L18 L19 | L2 A7 L3 L16 L19 A10 | L0 A5 L1 L4 L7 A8 | L0 A5 L1 L4 L5 L6 L7 | L1 A6 L2 L8 L9 L10 L11 | L1 A6 L2 L8 L11 A11 bodies 2
extrude "押し出し27" cut 4 faces at (-10.679, 59.6107, 22.5) (-9.668, 75.3003, 22.5) (9.541, 75.3364, 22.5) (10.532, 60.1803, 22.5) along direction (0, 0, -1) blind 1 on bodies 2 bodies 2
named bodies: "モータ取り付け台", "BLDC", "リアクションホイール", "磁気エンコーダ"
